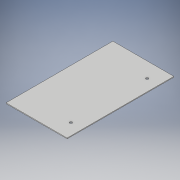
# Autodesk Inventor part: Plexiglass number plate 2
Saved by Autodesk Inventor 2019 (Build 230136000, 136)
## iProperties
Created: 2019-02-04
Part Number: Plexiglass number plate 2
Material: Generic
Document SubType Name: Modeling
Designer: mrhftc
Density: 1 g/cm^3
Appearance: Default
Author: mrhftc
Autodesk Inventor part; units mm, degrees
ref_plane "YZ Plane" through (0, 0, 0) normal (1, 0, 0) x (0, 1, 0)
ref_plane "XZ Plane" through (0, 0, 0) normal (0, 1, 0) x (-1, 0, 0)
ref_plane "XY Plane" through (0, 0, 0) normal (0, 0, 1) x (1, 0, 0)
sketch "Sketch1" plane through (0, 0, 0) normal (0, 1, 0) x (-1, 0, 0)
  line L0 (-68.8755, 120.8229) -> (-170.4755, 120.8229)
  line L1 (-170.4755, 120.8229) -> (-170.4755, -56.9771)
  line L2 (-170.4755, -56.9771) -> (-68.8755, -56.9771)
  line L3 (-68.8755, -56.9771) -> (-68.8755, 120.8229)
  circle A0 centre (-151.4255, 95.4229) radius 2.1
  circle A1 centre (-151.4255, -31.5771) radius 2.1
  point P0 (0, 0)
  dimension "d0" = 101.6
  dimension "d1" = 177.8
  dimension "d15" = 127
  dimension "d16" = 19.05
  dimension "d17" = 25.4
  constraints: 8 end point, 2 centre point, 2 parallel, 1 horizontal, 1 perpendicular
  measures "d0" distance between parallel lines of L1 L3
  measures "d1" distance between parallel lines of L2 L0
  measures "d15" distance of A0.centre A1.centre
  measures "d16" distance from line of L1 A1.centre
  measures "d17" distance from line of L0 A0.centre
extrude "Extrusion2" add sketch "Sketch1" along normal blind 1.27
body "Solid2"
